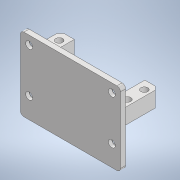
# Autodesk Inventor part: MotorCasingSmall
Saved by Autodesk Inventor 2022 (Build 260153000, 153)
## iProperties
Created: 2022-06-04
Part Number: MotorCasingSmall
Material: Generic
Document SubType Name: Modeling
Designer: frede
Density: 1 g/cm^3
Appearance: Default
Author: frede
Autodesk Inventor part; units mm, degrees
ref_plane "YZ Plane" through (0, 0, 0) normal (1, 0, 0) x (0, 1, 0)
ref_plane "XZ Plane" through (0, 0, 0) normal (0, 1, 0) x (-1, 0, 0)
ref_plane "XY Plane" through (0, 0, 0) normal (0, 0, 1) x (1, 0, 0)
sketch "Sketch1" plane through (0, 0, 0) normal (0, 0, 1) x (1, 0, 0)
  line L0 (-48.25, 32.55) -> (9.75, 32.55)
  line L1 (9.75, 32.55) -> (9.75, -10)
  line L2 (9.75, -10) -> (-48.25, -10)
  line L3 (-48.25, -10) -> (-48.25, 32.55)
  line L4 (-15.3, 32.55) -> (-3, 32.55) construction
  line L5 (-38.5, -4.8) -> (0, -4.8) construction
  line L6 (-3.7974, -7) -> (-34.7026, -7) construction
  line L7 (7.75, 21.3) -> (7.75, 23.7) construction
  line L8 (-46.25, 23.7) -> (-46.25, 21.3) construction
  point P0 (0, 0)
  point P1 (-48.25, 11.275)
  point P2 (9.75, 22.5)
  point P3 (-9.15, 32.55)
  dimension "d0" = 3
  dimension "d31" = 2
  dimension "d32" = 2
  constraints: 8 end point, 2 midpoint, 2 parallel, 2 point on line, 1 horizontal, 1 perpendicular
  measures "d0" distance between parallel lines of L6 L2
  measures "d31" distance between parallel lines of L7 L1
  measures "d32" distance between parallel lines of L8 L3
extrude "Extrusion1" add sketch "Sketch1" along normal blind 3
sketch "Sketch2" plane through (0, 0, 0) normal (0, 0, -1) x (-1, 0, 0)
  line L0 (-6.75, 21.3) -> (0, 21.3) construction
  line L1 (38.5, 21.3) -> (45.25, 21.3) construction
  line L2 (-0.7, 0) -> (-0.7, 20.8) construction
  line L3 (39.2, 0) -> (39.2, 20.8) construction
  line L4 (-0.7, 21.3) -> (-9.75, 21.3) construction
  line L5 (-9.75, 21.3) -> (-9.75, 11.3) construction
  line L6 (-9.75, 11.3) -> (-0.7, 11.3) construction
  line L7 (-0.7, 11.3) -> (-0.7, 21.3) construction
  line L8 (-9.75, -10) -> (-9.75, 32.55) construction
  line L9 (-1.2, 11.8) -> (-9.25, 11.8)
  line L10 (-9.25, 11.8) -> (-9.25, 20.8)
  line L11 (-9.25, 20.8) -> (-1.2, 20.8)
  line L12 (-1.2, 20.8) -> (-1.2, 11.8)
  line L13 (39.2, 21.3) -> (48.25, 21.3) construction
  line L14 (48.25, 21.3) -> (48.25, 11.3) construction
  line L15 (48.25, 11.3) -> (39.2, 11.3) construction
  line L16 (39.2, 11.3) -> (39.2, 21.3) construction
  line L17 (48.25, 32.55) -> (48.25, -10) construction
  line L18 (39.1953, -4.8086) -> (38, -7) construction
  line L19 (38, -7) -> (36, -7) construction
  line L20 (36, -7) -> (36, -9) construction
  line L21 (39.1953, -4.8086) -> (39.1953, -2.8086) construction
  line L22 (39.1953, -2.8086) -> (41.1953, -2.8086) construction
  line L23 (41.1953, -2.8086) -> (41.1953, -9) construction
  line L24 (41.1953, -9) -> (36, -9) construction
  line L25 (41.0953, -8.9) -> (41.0953, -2.9086)
  line L26 (41.0953, -2.9086) -> (39.2953, -2.9086)
  line L27 (39.2953, -2.9086) -> (39.2953, -4.8341)
  line L28 (39.2953, -4.8341) -> (38.0594, -7.1)
  line L29 (38.0594, -7.1) -> (36.1, -7.1)
  line L30 (36.1, -7.1) -> (36.1, -8.9)
  line L31 (36.1, -8.9) -> (41.0953, -8.9)
  line L32 (0.5, -7) -> (-0.6953, -4.8086) construction
  line L33 (-0.6953, -4.8086) -> (-0.6953, -2.8086) construction
  line L34 (-0.6953, -2.8086) -> (-2.6953, -2.8086) construction
  line L35 (0.5, -7) -> (2.5, -7) construction
  line L36 (2.5, -7) -> (2.5, -9) construction
  line L37 (2.5, -9) -> (-2.6953, -9) construction
  line L38 (-2.6953, -9) -> (-2.6953, -2.8086) construction
  line L39 (-2.5953, -8.9) -> (2.4, -8.9)
  line L40 (2.4, -8.9) -> (2.4, -7.1)
  line L41 (2.4, -7.1) -> (0.4406, -7.1)
  line L42 (0.4406, -7.1) -> (-0.7953, -4.8341)
  line L43 (-0.7953, -4.8341) -> (-0.7953, -2.9086)
  line L44 (-0.7953, -2.9086) -> (-2.5953, -2.9086)
  line L45 (-2.5953, -2.9086) -> (-2.5953, -8.9)
  line L46 (39.7, 11.8) -> (47.75, 11.8)
  line L47 (47.75, 11.8) -> (47.75, 20.8)
  line L48 (47.75, 20.8) -> (39.7, 20.8)
  line L49 (39.7, 20.8) -> (39.7, 11.8)
  point P0 (0, 0)
  point P1 (-0.7, 16.3)
  point P2 (-5.225, 21.3)
  point P3 (-9.75, 16.3)
  point P4 (39.2, 10.4)
  point P5 (43.725, 21.3)
  point P6 (48.25, 16.3)
  dimension "d3" = 10
  dimension "d4" = 0.5
  dimension "d5" = 10
  dimension "d7" = 2
  dimension "d8" = 2
  dimension "d9" = 2
  dimension "d10" = 2
  dimension "d11" = 0.1
  dimension "d12" = 2
  dimension "d13" = 2
  dimension "d14" = 2
  dimension "d15" = 2
  dimension "d16" = 0.1
  dimension "d59" = 0.5
  constraints: 88 end point, 20 perpendicular, 8 parallel, 6 midpoint, 6 point on line, 4 horizontal, 2 vertical, 22 other
  measures "d3" distance of L5.end L4.end
  measures "d4" distance between parallel lines of L6 L9
  measures "d5" distance of L13.end L14.end
  measures "d7" distance of L18.end L19.end
  measures "d8" distance of L19.end L20.end
  measures "d9" distance of L18.start L21.end
  measures "d10" distance of L21.end L22.end
  measures "d11" distance between parallel lines of L23 L25
  measures "d12" distance of L32.end L33.end
  measures "d13" distance of L33.end L34.end
  measures "d14" distance of L32.start L35.end
  measures "d15" distance of L35.end L36.end
  measures "d16" distance between parallel lines of L37 L39
  measures "d59" distance between parallel lines of L15 L46
ref_plane "Work Plane1" through (-45.25, 20.8, -19.7) normal (0, 0, -1) x (0, 1, 0)
extrude "Extrusion2" add sketch "Sketch2" along normal up to surface (19.7 mm away) contours L9 L10 L11 L12 | L49 L48 L47 L46
sketch "Sketch3" plane through (0, 0, 0) normal (0, 0, -1) x (-1, 0, 0)
  line L0 (-0.7, 0) -> (-0.7, 20.8) construction
  line L1 (39.2, 0) -> (39.2, 20.8) construction
  line L2 (-7.75, -10) -> (-7.75, 32.55) construction
  line L3 (46.25, 32.55) -> (46.25, -10) construction
  line L4 (39.1953, -4.8086) -> (38, -7) construction
  line L5 (38, -7) -> (36, -7) construction
  line L6 (36, -7) -> (36, -9) construction
  line L7 (39.1953, -4.8086) -> (39.1953, -2.8086) construction
  line L8 (39.1953, -2.8086) -> (41.1953, -2.8086) construction
  line L9 (41.1953, -2.8086) -> (41.1953, -9) construction
  line L10 (41.1953, -9) -> (36, -9) construction
  line L11 (41.0953, -8.9) -> (41.0953, -2.9086)
  line L12 (41.0953, -2.9086) -> (39.2953, -2.9086)
  line L13 (39.2953, -2.9086) -> (39.2953, -4.8341)
  line L14 (39.2953, -4.8341) -> (38.0594, -7.1)
  line L15 (38.0594, -7.1) -> (36.1, -7.1)
  line L16 (36.1, -7.1) -> (36.1, -8.9)
  line L17 (36.1, -8.9) -> (41.0953, -8.9)
  line L18 (0.5, -7) -> (-0.6953, -4.8086) construction
  line L19 (-0.6953, -4.8086) -> (-0.6953, -2.8086) construction
  line L20 (-0.6953, -2.8086) -> (-2.6953, -2.8086) construction
  line L21 (0.5, -7) -> (2.5, -7) construction
  line L22 (2.5, -7) -> (2.5, -9) construction
  line L23 (2.5, -9) -> (-2.6953, -9) construction
  line L24 (-2.6953, -9) -> (-2.6953, -2.8086) construction
  line L25 (-2.5953, -8.9) -> (2.4, -8.9)
  line L26 (2.4, -8.9) -> (2.4, -7.1)
  line L27 (2.4, -7.1) -> (0.4406, -7.1)
  line L28 (0.4406, -7.1) -> (-0.7953, -4.8341)
  line L29 (-0.7953, -4.8341) -> (-0.7953, -2.9086)
  line L30 (-0.7953, -2.9086) -> (-2.5953, -2.9086)
  line L31 (-2.5953, -2.9086) -> (-2.5953, -8.9)
  point P0 (0, 0)
  point P1 (0, 0)
  point P2 (-0.7, 16.3)
  point P3 (-7.75, 16.3)
  point P4 (39.2, 10.4)
  point P5 (46.25, 16.3)
  dimension "d19" = 2
  dimension "d20" = 2
  dimension "d21" = 2
  dimension "d22" = 2
  dimension "d23" = 0.1
  dimension "d24" = 2
  dimension "d25" = 2
  dimension "d26" = 2
  dimension "d27" = 2
  dimension "d28" = 0.1
  constraints: 64 end point, 16 perpendicular, 3 point on line, 2 horizontal, 2 vertical, 1 midpoint, 16 other
  measures "d19" distance of L4.end L5.end
  measures "d20" distance of L5.end L6.end
  measures "d21" distance of L7.start L8.start
  measures "d22" distance of L8.start L8.end
  measures "d23" distance between parallel lines of L9 L11
  measures "d24" distance of L18.end L20.start
  measures "d25" distance of L20.start L20.end
  measures "d26" distance of L18.start L21.end
  measures "d27" distance of L21.end L23.start
  measures "d28" distance between parallel lines of L23 L25
extrude "Extrusion3" add sketch "Sketch3" along normal blind 4
sketch "Sketch4" plane through (1.2, 20.8, 0) normal (0, 1, 0) x (1, 0, 0)
  arc A0 (5.9164, 16.0673) -> (5.9164, 13.4827) centre (4.2611, 14.775) ccw construction
  arc A1 (5.9164, 6.2173) -> (5.9164, 3.6327) centre (4.2611, 4.925) ccw construction
  arc A2 (-46.8164, 3.6327) -> (-46.8164, 6.2173) centre (-45.1611, 4.925) ccw construction
  arc A3 (-46.8164, 13.4827) -> (-46.8164, 16.0673) centre (-45.1611, 14.775) ccw construction
  circle A4 centre (-45.1611, 14.775) radius 2
  circle A5 centre (-45.1611, 4.925) radius 2
  circle A6 centre (4.2611, 14.775) radius 2
  circle A7 centre (4.2611, 4.925) radius 2
  point P0 (-1.2, 0)
  dimension "d45" = 4
  dimension "d46" = 4
  dimension "d47" = 4
  dimension "d48" = 4
  constraints: 4 centre point, 4 coincident
  measures "d45" diameter of A4
  measures "d46" diameter of A5
  measures "d47" diameter of A6
  measures "d48" diameter of A7
sketch "Sketch5" plane through (0, 0, 0) normal (0, 0, -1) x (-1, 0, 0)
  circle A0 centre (-4.75, 27.55) radius 2
  circle A1 centre (-4.75, 2) radius 2
  circle A2 centre (43.25, 2) radius 2
  circle A3 centre (43.25, 27.55) radius 2
  line L0 (48.25, 32.55) -> (48.25, -10) projected
  line L1 (-9.75, 32.55) -> (48.25, 32.55) projected
  line L2 (48.25, -10) -> (-9.75, -10) projected
  line L3 (-9.75, -10) -> (-9.75, 32.55) projected
  point P0 (0, 0)
  dimension "d33" = 4
  dimension "d34" = 4
  dimension "d35" = 4
  dimension "d36" = 4
  dimension "d37" = 5
  dimension "d38" = 5
  dimension "d39" = 12
  dimension "d58" = 5
  constraints: 4 centre point, 2 horizontal alignment, 2 vertical alignment
  measures "d33" diameter of A0
  measures "d34" diameter of A1
  measures "d35" diameter of A2
  measures "d36" diameter of A3
  measures "d37" distance from line of L0 A3.centre
  measures "d38" distance from line of L1 A3.centre
  measures "d39" distance from line of L2 A2.centre
  measures "d58" distance from line of L3 A0.centre
extrude "Extrusion4" cut sketch "Sketch5" against normal through all contours A0 | A1 | A2 | A3
chamfer "Chamfer1" distance 1 angle 45 4 edges at (6.75, 27.55, 0) (6.75, 2, 0) (-41.25, 2, 0) (-41.25, 27.55, 0)
extrude "Extrusion5" cut sketch "Sketch4" against normal through all
chamfer "Chamfer2" distance 2 angle 45 2 edges at (9.25, 16.3, -19.7) (-47.75, 16.3, -19.7)
fillet "Fillet1" radius 2 4 edges at (9.75, -10, 1.5) (9.75, 32.55, 1.5) (-48.25, 32.55, 1.5) (-48.25, -10, 1.5)
chamfer "Chamfer3" distance 2 angle 45 2 edges at (-41.0953, -8.9, -2) (2.5953, -8.9, -2)
body "Solid1"
